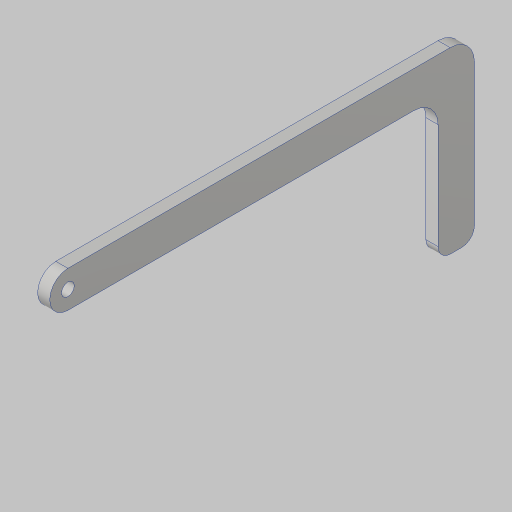
# Autodesk Inventor part: CHD-002
Saved by Autodesk Inventor 2023.5 (Build 275446000, 446)
## iProperties
Created: 2025-02-02
Part Number: CHD-002
Material: Aluminum 6061
Document SubType Name: Modeling
Designer: slick
Density: 2.7 g/cm^3
Appearance: Aluminum - Flat
Author: slick
Autodesk Inventor part; units mm, degrees
ref_plane "YZ Plane" through (0, 0, 0) normal (1, 0, 0) x (0, 1, 0)
ref_plane "XZ Plane" through (0, 0, 0) normal (0, 1, 0) x (-1, 0, 0)
ref_plane "XY Plane" through (0, 0, 0) normal (0, 0, 1) x (1, 0, 0)
sketch "Sketch1" plane through (0, 0, 0) normal (1, 0, 0) x (0, 1, 0)
  line L0 (0, 0) -> (50.8, 0) construction
  line L1 (50.8, 0) -> (50.8, -25.4) construction
  line L2 (50.8, -25.4) -> (0, -25.4) construction
  line L3 (0, -25.4) -> (0, 0) construction
  line L4 (12.7, -25.4) -> (139.7, -25.4) construction
  line L5 (139.7, -25.4) -> (139.7, -111.252) construction
  line L6 (139.7, -111.252) -> (12.7, -111.252) construction
  line L7 (12.7, -111.252) -> (12.7, -25.4) construction
  line L8 (80.9625, -111.252) -> (665.1625, -111.252) construction
  line L9 (665.1625, -111.252) -> (665.1625, -320.802) construction
  line L10 (665.1625, -320.802) -> (80.9625, -320.802) construction
  line L11 (80.9625, -320.802) -> (80.9625, -111.252) construction
  point P0 (0, -12.7)
  dimension "d0" = 50.8
  dimension "d1" = 25.4
  dimension "d2" = 12.7
  dimension "d3" = 85.852
  dimension "d4" = 127
  dimension "d5" = 80.9625
  dimension "d6" = 209.55
  dimension "d7" = 584.2
  constraints: 24 end point, 6 parallel, 3 horizontal, 3 perpendicular, 2 point on line, 1 midpoint
  measures "d0" distance of L1.end L2.end
  measures "d1" distance of L0.end L1.end
  measures "d2" distance between parallel lines of L3 L7
  measures "d3" distance of L4.end L5.end
  measures "d4" distance of L5.end L6.end
  measures "d5" distance from line of L11 point (0, -12.7)
  measures "d6" distance of L8.end L9.end
  measures "d7" distance of L8.start L8.end
sketch "Sketch2" plane through (0, 0, 0) normal (1, 0, 0) x (0, 1, 0)
  line L0 (139.7, -25.4) -> (139.7, -111.252) construction
  line L1 (80.9625, -320.802) -> (80.9625, -111.252) construction
  line L2 (139.7, -111.252) -> (12.7, -111.252) construction
  line L3 (50.8, 0) -> (50.8, -25.4) construction
  line L4 (12.7, -25.4) -> (139.7, -25.4) construction
  line L5 (12.7, -111.252) -> (12.7, -25.4) construction
  line L6 (50.8, -25.4) -> (0, -25.4) construction
  line L7 (0, -25.4) -> (0, 0) construction
  line L8 (0, 0) -> (50.8, 0) construction
  line L9 (665.1625, -320.802) -> (80.9625, -320.802) construction
  line L10 (80.9625, -111.252) -> (665.1625, -111.252) construction
  line L11 (665.1625, -111.252) -> (665.1625, -320.802) construction
  line L12 (50.8, -25.4) -> (190.5, -25.4) construction
  line L13 (190.5, -25.4) -> (190.5, 0) construction
  line L14 (190.5, 0) -> (50.8, 0) construction
  line L15 (50.8, 0) -> (50.8, -25.4) construction
  line L16 (165.1, -12.7) -> (165.1, -216.027) construction
  line L17 (165.1, -216.027) -> (80.9625, -216.027) construction
  line L18 (80.9625, -225.552) -> (174.625, -225.552)
  line L19 (174.625, -225.552) -> (174.625, -12.7)
  line L20 (80.9625, -206.502) -> (155.575, -206.502)
  line L21 (155.575, -206.502) -> (155.575, -12.7)
  line L22 (80.9625, -206.502) -> (80.9625, -225.552)
  arc A0 (174.625, -12.7) -> (155.575, -12.7) centre (165.1, -12.7) ccw
  point P0 (0, -12.7)
  point P1 (190.5, -12.7)
  dimension "d8" = 50.8
  dimension "d9" = 25.4
  dimension "d10" = 9.525
  dimension "d11" = 9.525
  dimension "d12" = 139.7
  constraints: 22 end point, 5 perpendicular, 3 horizontal alignment, 2 midpoint, 2 parallel, 2 point on circle, 2 point on line, 1 centre point, 1 coincident, 1 collinear, 1 horizontal, 2 other
  measures "d8" distance between parallel lines of L0 L13
  measures "d9" distance from line of L0 L16.start
  measures "d10" distance between parallel lines of L17 L18
  measures "d11" distance between parallel lines of L17 L20
  measures "d12" distance between parallel lines of L3 L13
extrude "Extrusion1" add sketch "Sketch2" along normal blind 6.35
fillet "Fillet1" radius 12.7 2 edges at (3.175, 155.575, -206.502) (3.175, 174.625, -225.552)
fillet "Fillet2" radius 6.604 2 edges at (3.175, 80.9625, -225.552) (3.175, 80.9625, -206.502)
hole "Hole1" at (0, 139.7, -111.252) at (0, 139.7, -25.4) at (0, 80.9625, -111.252) at (0, 80.9625, -320.802) at (0, 50.8, -25.4) at (0, 12.7, -111.252) at (0, 50.8, 0) at (0, 0, -25.4) at (0, 0, -12.7) at (0, 165.1, -12.7) direction (1, 0, 0) diameter 6.7564 end through all clearance for "Flat Head Machine Screw (82)" size "1/4" standard "Ansi Unified Screw Threads"
body "Solid1"
